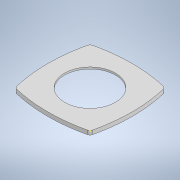
# Autodesk Inventor part: Boat Handle (Handle) Rev A
Saved by Autodesk Inventor 2021 (Build 250183000, 183)
## iProperties
Created: 2020-09-03
Part Number: Boat Handle (Handle) Rev A
Material: Generic
Document SubType Name: Modeling
Designer: cmzgt
Density: 1 g/cm^3
Appearance: Default
Author: cmzgt
## iProperties of the stored document _3DPrint.ipt
Created: 2020-09-03
Part Number: _3DPrint
Material: Generic
Document SubType Name: Modeling
Designer: cmzgt
Density: 1 g/cm^3
Appearance: Default
Author: cmzgt
Autodesk Inventor part; units mm, degrees
ref_plane "YZ Plane" through (0, 0, 0) normal (1, 0, 0) x (0, 1, 0)
ref_plane "XZ Plane" through (0, 0, 0) normal (0, 1, 0) x (-1, 0, 0)
ref_plane "XY Plane" through (0, 0, 0) normal (0, 0, 1) x (1, 0, 0)
sketch "Sketch1" plane through (0, 0, 0) normal (0, 1, 0) x (-1, 0, 0)
  line L0 (0, 0) -> (0, -71.12)
  line L1 (0, -71.12) -> (71.12, -71.12)
  line L2 (71.12, -71.12) -> (71.12, 0)
  line L3 (71.12, 0) -> (0, 0)
  arc A0 (71.12, -71.12) -> (71.12, 0) centre (-71.8439, -35.56) ccw
  arc A1 (0, 0) -> (0, -71.12) centre (142.9639, -35.56) ccw
  arc A2 (0, -71.12) -> (71.12, -71.12) centre (35.56, 71.8439) ccw
  arc A3 (71.12, 0) -> (0, 0) centre (35.56, -142.9639) ccw
  circle A4 centre (35.56, -35.56) radius 24.13
  dimension "d9" = 71.12
  dimension "d10" = 71.12
  dimension "d14" = 147.32
  dimension "d17" = 48.26
  dimension "d18" = 35.56
  dimension "d19" = 35.56
  constraints: 8 end point, 8 point on circle, 5 centre point, 3 equal radius, 3 perpendicular, 1 vertical
  measures "d9" distance of L0.start L0.end
  measures "d10" distance of L0.end L1.end
  measures "d14" radius of A3
  measures "d17" diameter of A4
  measures "d18" distance from line of A4.centre L0
  measures "d19" distance from line of A4.centre L1
extrude "Extrusion1" add sketch "Sketch1" along normal blind 3.81
fillet "Fillet1" radius 3.175 4 edges at (0, 1.905, 0) (0, 1.905, -71.12) (-71.12, 1.905, 0) (-71.12, 1.905, -71.12)
sketch "Sketch2" plane through (0, 3.81, 0) normal (0, 1, 0) x (1, 0, 0)
  point P0 (0, 0)
sketch "Sketch3" plane through (0, 0, 0) normal (0, -1, 0) x (1, 0, 0)
  circle A0 centre (-35.56, -35.56) radius 24.13 projected
  circle A1 centre (-35.56, -35.56) radius 31.623
  circle A2 centre (-35.56, -35.56) radius 24.13
  point P0 (0, 0)
  dimension "d23" = 63.246
  constraints: 2 centre point, 2 coincident
  measures "d23" diameter of A1
extrude "Extrusion2" cut sketch "Sketch3" against normal blind 2.1079
body "Solid1"
